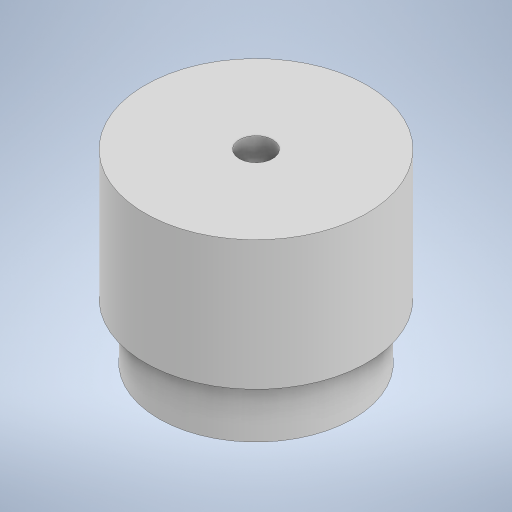
# Autodesk Inventor part: tapon optica SiPM
Saved by Autodesk Inventor 2024.2 (Build 282272000, 272)
## iProperties
Created: 2026-02-13
Part Number: tapon optica SiPM
Material: Generic
Document SubType Name: Modeling
Designer: ja.restrepo1
Density: 1 g/cm^3
Appearance: Default
Author: ja.restrepo1
Autodesk Inventor part; units mm, degrees
ref_plane "YZ Plane" through (0, 0, 0) normal (1, 0, 0) x (0, 1, 0)
ref_plane "XZ Plane" through (0, 0, 0) normal (0, 1, 0) x (-1, 0, 0)
ref_plane "XY Plane" through (0, 0, 0) normal (0, 0, 1) x (1, 0, 0)
sketch "Sketch1" plane through (0, 0, 0) normal (1, 0, 0) x (0, 1, 0)
  line L0 (10, -0.9) -> (7, -0.9)
  line L1 (0, -0.9) -> (0, -3.8713) construction
  line L2 (0, -5.25) -> (3, -5.25)
  line L3 (3, -5.25) -> (3, -6)
  line L4 (3, -6) -> (10, -6)
  line L5 (10, -6) -> (10, -0.9)
  line L6 (10, 0) -> (0, 0) construction
  line L7 (-2, 0) -> (12, 0) projected
  line L8 (7, -0.9) -> (0, -3.8713)
  line L9 (7, -0.9) -> (0, -0.9) construction
  line L10 (0, -3.8713) -> (0, -5.25)
  point P0 (0, -4.5607)
  point P1 (5, 0)
  dimension "d2" = 6
  dimension "d3" = 5.25
  dimension "d4" = 7
  dimension "d9" = 3
  dimension "d10" = 157
  dimension "d11" = 0.9
  dimension "d12" = 10
  dimension "d13" = 5
  constraints: 20 end point, 9 perpendicular, 3 horizontal, 2 midpoint, 2 vertical alignment, 1 coincident, 1 horizontal alignment
  measures "d2" distance between parallel lines of L4 L6
  measures "d3" distance between parallel lines of L6 L2
  measures "d4" distance of L3.end L4.end
  measures "d9" distance of L0.end L0.start
  measures "d10" angle of L0 L8
  measures "d11" distance between parallel lines of L6 L0
  measures "d12" distance between parallel lines of L10 L5
  measures "d13" distance of point (0, 0) point (5, 0)
revolve "Revolution1" add sketch "Sketch1" angle 360 about axis through (0, -10, 0) along (0, 1, 0)
fillet "Fillet1" radius 0.2 1 edges at (0, 3, 5.25)
fillet "Fillet2" radius 0.36 1 edges at (0, 0, 3.8713)
body "Solid1"
